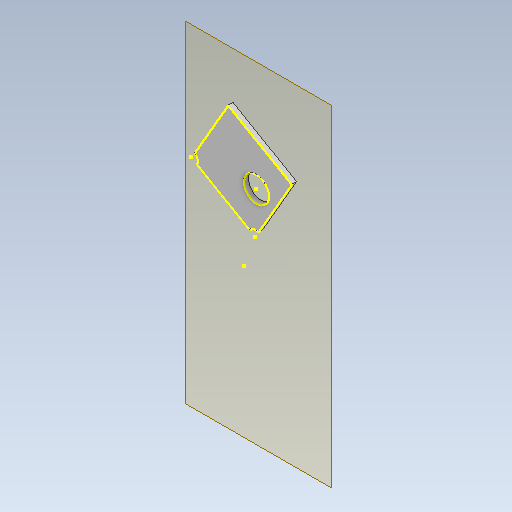
# Autodesk Inventor part: wooden_internal
Saved by Autodesk Inventor 2020 (Build 240168000, 168)
## iProperties
Created: 2019-07-29
Part Number: wooden_internal
Material: Generic
Document SubType Name: Modeling
Designer: erwin
Density: 1 g/cm^3
Appearance: Default
Author: erwin
Autodesk Inventor part; units mm, degrees
ref_plane "YZ Plane" through (0, 0, 0) normal (1, 0, 0) x (0, 1, 0)
ref_plane "XZ Plane" through (0, 0, 0) normal (0, 1, 0) x (-1, 0, 0)
ref_plane "XY Plane" through (0, 0, 0) normal (0, 0, 1) x (1, 0, 0)
ref_plane "Work Plane1" through (0, 0, 0) normal (0, 0, 1) x (1, 0, 0)
sketch "Sketch1" plane through (0, 0, 0) normal (0, 0, 1) x (1, 0, 0)
  circle A0 centre (68.259454, 214.654052) radius 4
  line L0 (64.259454, -185.345948) -> (64.259454, -225.345948)
  arc A1 (72.259454, -185.345948) -> (64.259454, -185.345948) centre (68.259454, -185.345948) ccw
  line L1 (72.259454, -225.345948) -> (72.259454, -185.345948)
  arc A2 (64.259454, -225.345948) -> (72.259454, -225.345948) centre (68.259454, -225.345948) ccw
  line L2 (-101.259454, 230.542101) -> (-90.867149, 224.542101)
  line L3 (-90.867149, 224.542101) -> (-108.867149, 193.365186)
  line L4 (-108.867149, 193.365186) -> (-119.259454, 199.365186)
  line L5 (-137.259454, 168.188271) -> (-119.259454, 199.365186)
  line L6 (-137.259454, 168.188271) -> (-106.082539, 150.188271)
  line L7 (-106.082539, 150.188271) -> (-112.082539, 139.795967)
  line L8 (-80.905625, 121.795967) -> (-112.082539, 139.795967)
  line L9 (-80.905625, 121.795967) -> (-74.905625, 132.188271)
  line L10 (-74.905625, 132.188271) -> (-43.72871, 114.188271)
  line L11 (-43.72871, 114.188271) -> (-49.72871, 103.795967)
  line L12 (-18.551796, 85.795967) -> (-49.72871, 103.795967)
  line L13 (-18.551796, 85.795967) -> (-12.551796, 96.188271)
  line L14 (-12.551796, 96.188271) -> (18.625119, 78.188271)
  line L15 (18.625119, 78.188271) -> (12.625119, 67.795967)
  line L16 (23.259454, 61.656231) -> (12.625119, 67.795967)
  line L17 (23.259454, -7.001047) -> (23.259454, 61.656231)
  line L18 (23.259454, -7.001047) -> (35.259454, -7.001047)
  line L19 (35.259454, -7.001047) -> (35.259454, -43.001047)
  line L20 (35.259454, -43.001047) -> (23.259454, -43.001047)
  line L21 (23.259454, -79.001047) -> (23.259454, -43.001047)
  line L22 (23.259454, -79.001047) -> (35.259454, -79.001047)
  line L23 (35.259454, -79.001047) -> (35.259454, -115.001047)
  line L24 (35.259454, -115.001047) -> (23.259454, -115.001047)
  line L25 (23.259454, -151.001047) -> (23.259454, -115.001047)
  line L26 (23.259454, -151.001047) -> (35.259454, -151.001047)
  line L27 (35.259454, -151.001047) -> (35.259454, -187.001047)
  line L28 (35.259454, -187.001047) -> (23.259454, -187.001047)
  line L29 (23.259454, -223.001047) -> (23.259454, -187.001047)
  line L30 (23.259454, -223.001047) -> (35.259454, -223.001047)
  line L31 (35.259454, -223.001047) -> (35.259454, -259.001047)
  line L32 (35.259454, -259.001047) -> (23.259454, -259.001047)
  line L33 (23.259454, -295.001047) -> (23.259454, -259.001047)
  line L34 (23.259454, -295.001047) -> (35.259454, -295.001047)
  line L35 (35.259454, -295.001047) -> (35.259454, -331.001047)
  line L36 (105.759454, -290.297853) -> (35.259454, -331.001047)
  arc A3 (105.759454, -290.297853) -> (143.259454, -225.345948) centre (68.259454, -225.345948) ccw
  line L37 (143.259454, -185.345948) -> (143.259454, -225.345948)
  arc A4 (143.259454, -185.345948) -> (125.301159, -136.650529) centre (68.259454, -185.345948) ccw
  arc A5 (114.658634, -107.792431) -> (125.301159, -136.650529) centre (159.105469, -107.792431) ccw
  line L38 (114.658634, 129.266291) -> (114.658634, -107.792431)
  arc A6 (128.128133, 169.479488) -> (114.658634, 129.266291) centre (181.421641, 129.266291) ccw
  arc A7 (128.128133, 169.479488) -> (62.965391, 289.466971) centre (68.259454, 214.654052) ccw
  arc A8 (5.90664, 302.61499) -> (62.965391, 289.466971) centre (55.90664, 389.21753) ccw
  line L39 (-43.259454, 331.001047) -> (5.90664, 302.61499)
  line L40 (-65.259454, 292.89593) -> (-43.259454, 331.001047)
  line L41 (-65.259454, 292.89593) -> (-54.867149, 286.89593)
  line L42 (-54.867149, 286.89593) -> (-72.867149, 255.719015)
  line L43 (-72.867149, 255.719015) -> (-83.259454, 261.719015)
  line L44 (-101.259454, 230.542101) -> (-83.259454, 261.719015)
  circle A9 centre (28.259454, 174.654052) radius 30
  line L45 (71.945627, 130.542101) -> (61.553322, 136.542101)
  line L46 (61.553322, 136.542101) -> (79.553322, 167.719015)
  line L47 (79.553322, 167.719015) -> (89.945627, 161.719015)
  line L48 (89.945627, 161.719015) -> (71.945627, 130.542101)
  line L49 (-32.867149, 325.001047) -> (-54.867149, 286.89593)
  line L50 (61.553322, 136.542101) -> (30.062941, 81.999161)
  line L51 (-12.551796, 96.188271) -> (18.625119, 78.188271)
  line L52 (-38.001123, 314.108743) -> (112.687297, 227.108743)
  line L53 (-54.867149, 286.89593) -> (-72.867149, 255.719015)
  line L54 (-74.905625, 132.188271) -> (-43.72871, 114.188271)
  line L55 (-38.001123, 314.108743) -> (112.687297, 227.108743)
  line L56 (119.553322, 237.001047) -> (79.553322, 167.719015)
  line L57 (-38.867149, 314.608743) -> (-126.867149, 162.188271)
  line L58 (-126.867149, 162.188271) -> (25.553322, 74.188271)
  line L59 (25.553322, 74.188271) -> (113.553322, 226.608743)
  line L60 (113.553322, 226.608743) -> (-38.867149, 314.608743)
  circle A10 centre (-126.867149, 162.188271) radius 15
  circle A11 centre (25.553322, 74.188271) radius 15
  circle A12 centre (28.259454, 174.654052) radius 30
  point P0 (0, 0)
  point P1 (37.343087, 270.608743)
  point P2 (37.343087, 270.608743)
  point P3 (70.553322, 152.130558)
  point P4 (-59.317167, 123.188271)
  point P5 (12.562941, 81.688271)
  point P6 (33.053322, 87.178653)
  point P7 (-119.367149, 175.178653)
  point P8 (-113.876768, 154.688271)
  dimension "d0" = 30
  dimension "d1" = 30
  dimension "d2" = 60
  constraints: 8 end point, 5 midpoint, 3 centre point, 3 coincident, 2 perpendicular, 2 point on line, 1 collinear, 1 parallel
  measures "d0" diameter of A10
  measures "d1" diameter of A11
  measures "d2" diameter of A12
extrude "Extrusion1" add sketch "Sketch1" along normal blind 12 contours A0 | L57 L42 L49 L60 L52 L56 L46 L50 A11 L14 L58 L10 L6 A10 L3
move faces "Move1" translate (-0.5, -0.866025, 0) faces at (62.457823, 256.108743, 4)
sketch "Sketch2" plane through (0, 0, 12) normal (0, 0, 1) x (1, 0, 0)
  line L0 (-39.367149, 313.742717) -> (-119.367149, 175.178653)
  arc A0 (-113.876768, 154.688271) -> (-119.367149, 175.178653) centre (-126.867149, 162.188271) ccw
  line L1 (-113.876768, 154.688271) -> (12.562941, 81.688271)
  arc A1 (33.053322, 87.178653) -> (12.562941, 81.688271) centre (25.553322, 74.188271) ccw
  line L2 (33.053322, 87.178653) -> (113.053322, 225.742717)
  line L3 (113.053322, 225.742717) -> (-39.367149, 313.742717)
  circle A2 centre (28.259454, 174.654052) radius 30
  point P0 (0, 0)
equation "\"d1\" = d0"
body "Solid1"
